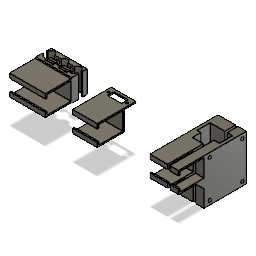
Expanded Dock v9 (Autodesk Fusion 360 design; units mm, degrees)
Autodesk Fusion 360 part; units mm, degrees
(part 1 of 2)
sketch "Sketch1" plane through (0, 0, 0) normal (1, 0, 0) x (0, 0, -1)
  line L0 (0, 0) -> (27, 0)
  line L1 (27, 0) -> (27, 60)
  line L2 (27, 60) -> (0, 60)
  line L3 (0, 60) -> (0, 0)
  dimension "d1" = 60
  dimension "d2" = 27
  constraint horizontal L0
  constraint vertical L1
  constraint horizontal L2
  constraint vertical L3
  constraint coincident L0.start L3.end
  measures "d1" distance of L0.start L2.end
  measures "d2" distance of L0.start L0.end
  measures "d70" distance of L0.end
  measures "d79" distance of L0.end
extrude "Extrude1" add sketch "Sketch1" along normal blind 2 makes body 1
sketch "Sketch2" plane through (2, 0, 0) normal (1, 0, 0) x (0, 0, -1)
  line L0 (0, 60) -> (0, 0)
  line L1 (0, 0) -> (27, 0)
  line L2 (27, 0) -> (27, 60)
  line L3 (27, 60) -> (0, 60)
  line L4 (0, 60) -> (11, 60)
  line L5 (11, 60) -> (11, 39)
  line L6 (11, 39) -> (0, 39)
  line L7 (0, 39) -> (0, 60)
  dimension "d5" = 21
  dimension "d6" = 11
  constraint horizontal L4
  constraint vertical L5
  constraint horizontal L6
  constraint vertical L7
  constraint coincident L0.start L3.end
  measures "d5" distance of L0.start L6.end
  measures "d6" distance of L0.start L4.end
extrude "Extrude2" add sketch "Sketch2" along normal blind 5 contours L0 L3 L4 L5 L6 L7 bodies 1
sketch "Sketch3" plane through (2, 0, 0) normal (1, 0, 0) x (0, 0, -1)
  line L0 (11, 60) -> (11, 39)
  line L1 (11, 39) -> (0, 39)
  line L2 (27, 0) -> (27, 60)
  line L3 (27, 60) -> (11, 60)
  line L4 (27, 0) -> (23, 0)
  line L5 (23, 0) -> (23, 20)
  line L6 (23, 20) -> (27, 20)
  line L7 (27, 20) -> (27, 0)
  line L8 (0, 0) -> (2, 0)
  line L9 (2, 0) -> (2, 20)
  line L10 (2, 20) -> (0, 20)
  line L11 (0, 20) -> (0, 0)
  dimension "d11" = 20
  dimension "d12" = 4
  dimension "d13" = 20
  dimension "d14" = 2
  constraint horizontal L4
  constraint vertical L5
  constraint horizontal L6
  constraint vertical L7
  constraint coincident L2.start L4.start
  constraint horizontal L8
  constraint vertical L9
  constraint horizontal L10
  constraint vertical L11
  constraint coincident L8.start L11.end
  measures "d11" distance of L2.start L6.end
  measures "d12" distance of L2.start L4.end
  measures "d13" distance of L8.start L10.end
  measures "d14" distance of L8.start L8.end
extrude "Extrude3" add sketch "Sketch3" along normal blind 27 bodies 1
sketch "Sketch4" plane through (0, 0, 0) normal (0, 0, 1) x (1, 0, 0)
  line L0 (0, 60) -> (0, 0)
  line L1 (0, 0) -> (29, 0)
  line L2 (29, 0) -> (29, 20)
  line L3 (29, 20) -> (2, 20)
  line L4 (2, 20) -> (2, 39)
  line L5 (2, 39) -> (7, 39)
  line L6 (7, 39) -> (7, 60)
  line L7 (7, 60) -> (0, 60)
  line L8 (0, 0) -> (29, 0)
  line L9 (29, 0) -> (29, 60)
  line L10 (29, 60) -> (0, 60)
  line L11 (0, 60) -> (0, 0)
  dimension "d17" = 29
  constraint horizontal L8
  constraint vertical L9
  constraint horizontal L10
  constraint vertical L11
  constraint coincident L0.end L1.start
  measures "d17" distance of L0.end L1.end
extrude "Extrude4" add sketch "Sketch4" along normal blind 5 bodies 1
sketch "Sketch5" plane through (0, 0, -27) normal (0, 0, -1) x (-1, 0, 0)
  line L0 (0, 0) -> (0, 60)
  line L1 (0, 60) -> (-2, 60)
  line L2 (-2, 60) -> (-2, 20)
  line L3 (-2, 20) -> (-29, 20)
  line L4 (-29, 20) -> (-29, 0)
  line L5 (-29, 0) -> (0, 0)
  line L6 (0, 0) -> (-29, 0)
  line L7 (-29, 0) -> (-29, 60)
  line L8 (-29, 60) -> (0, 60)
  line L9 (0, 60) -> (0, 0)
  dimension "d20" = 29
  constraint horizontal L6
  constraint vertical L7
  constraint horizontal L8
  constraint vertical L9
  constraint coincident L0.start L5.end
  measures "d20" distance of L0.start L4.end
extrude "Extrude5" add sketch "Sketch5" along normal blind 2 bodies 1
extrude "Extrude6" add 1 faces at (9.6667, 20, -29) along direction (0, 0, -1) blind 3 on bodies 1 bodies 1
sketch "Sketch6" plane through (29, 0, 0) normal (1, 0, 0) x (0, 0, -1)
  line L0 (-5, 0) -> (2, 0)
  line L1 (2, 0) -> (2, 20)
  line L2 (2, 20) -> (0, 20)
  line L3 (0, 20) -> (0, 60)
  line L4 (0, 60) -> (-5, 60)
  line L5 (-5, 60) -> (-5, 0)
  line L6 (32, 0) -> (-5, 0)
  line L7 (-5, 0) -> (-5, 60)
  line L8 (-5, 60) -> (32, 60)
  line L9 (32, 60) -> (32, 0)
  line L10 (32, 0) -> (32, 60)
  line L11 (23, 0) -> (27, 0)
  line L12 (27, 0) -> (27, 20)
  line L13 (27, 20) -> (23, 20)
  line L14 (23, 20) -> (23, 0)
  line L15 (27, 60) -> (32, 60)
  line L16 (32, 60) -> (32, 0)
  line L17 (32, 0) -> (27, 0)
  line L18 (27, 0) -> (27, 60)
  point P0 (23, 0)
  point P1 (27, 20)
  point P2 (27, 60)
  constraint horizontal L6
  constraint vertical L7
  constraint horizontal L8
  constraint vertical L9
  constraint coincident L4.end L5.start
  constraint coincident L6.start L10
  constraint horizontal L11
  constraint vertical L12
  constraint horizontal L13
  constraint vertical L14
  constraint coincident P1 L12.end
  constraint coincident P0 L11.start
  constraint horizontal L15
  constraint vertical L16
  constraint horizontal L17
  constraint vertical L18
  constraint coincident L6.start L9.end
  constraint coincident P2 L15.start
extrude "Extrude7" add sketch "Sketch6" along normal blind 5 separate body contours L0 L1 L2 L3 L4 L5 L6 L7 L8 | L6 L11 L12 L13 L14 L18 | L6 L8 L9 L10 L12 L15 L16 L17 L18 makes body 2 at (29, 6.6667, 1) makes body 3 at (29, 6.6667, -27.3333)
sketch "Sketch7" plane through (34, 0, 0) normal (1, 0, 0) x (0, 0, -1)
  line L0 (2, 0) -> (2, 20)
  line L1 (2, 20) -> (0, 20)
  line L2 (0, 20) -> (0, 60)
  line L3 (0, 60) -> (-5, 60)
  line L4 (-5, 60) -> (-5, 0)
  line L5 (-5, 0) -> (2, 0)
  line L6 (32, 0) -> (-5, 0)
  line L7 (-5, 0) -> (-5, 60)
  line L8 (-5, 60) -> (32, 60)
  line L9 (32, 60) -> (32, 0)
  point P0 (32, 0)
  constraint horizontal L6
  constraint vertical L7
  constraint horizontal L8
  constraint vertical L9
  constraint coincident L3.end L4.start
  constraint coincident P0 L6.start
extrude "Extrude8" add sketch "Sketch7" along normal blind 1 bodies 2 3
extrude "Extrude9" cut 2 faces at (29, 6.6667, -27.3333) (29, 6.6667, 1) along direction (-1, 0, 0) blind 1 on bodies 1 bodies 1
extrude "Extrude10" cut 2 faces at (28, 6.6667, -27.3333) (28, 6.6667, 1) along direction (-1, 0, 0) blind 5 on bodies 1 bodies 1
extrude "Extrude11" add 2 faces at (29, 6.6667, -27.3333) (29, 6.6667, 1) along direction (-1, 0, 0) blind 1 on bodies 2 bodies 2
extrude "Extrude12" add 1 faces at (34, 46.6667, -16.6667) along direction (-1, 0, 0) blind 5 on bodies 2 bodies 2
sketch "Sketch8" plane through (7, 0, 0) normal (1, 0, 0) x (0, 0, -1)
  line L0 (0, 39) -> (11, 39)
  line L1 (11, 39) -> (11, 60)
  line L2 (11, 60) -> (0, 60)
  line L3 (0, 60) -> (0, 39)
extrude "Extrude13" add sketch "Sketch8" along normal blind 17 and the other way blind -22 bodies 2
extrude "Extrude14" add 2 faces at (28, 6.6667, 1) (28, 6.6667, -27.3333) along direction (-1, 0, 0) blind 4 on bodies 2 bodies 2
extrude "Extrude15" cut 2 faces at (23, 6.6667, 1) (23, 6.6667, -27.3333) along direction (-1, 0, 0) blind 2 on bodies 1 bodies 1
extrude "Extrude16" cut 1 faces at (29, 39.6667, -21.6667) along direction (1, 0, 0) blind 2 on bodies 2 bodies 2
sketch "Sketch9" plane through (31, 0, 0) normal (-1, 0, 0) x (0, 0, 1)
  line L0 (0, 39) -> (-11, 39)
  line L1 (-11, 39) -> (-11, 60)
  line L2 (-11, 60) -> (-27, 60)
  line L3 (-27, 60) -> (-27, 20)
  line L4 (-27, 20) -> (-23, 20)
  line L5 (-23, 20) -> (-23, 0)
  line L6 (-23, 0) -> (-2, 0)
  line L7 (-2, 0) -> (-2, 20)
  line L8 (-2, 20) -> (0, 20)
  line L9 (0, 20) -> (0, 39)
  line L10 (-23, 20) -> (-2, 20)
  line L11 (-2, 20) -> (-2, 0)
  line L12 (-2, 0) -> (-23, 0)
  line L13 (-23, 0) -> (-23, 20)
  constraint horizontal L10
  constraint vertical L11
  constraint horizontal L12
  constraint vertical L13
  constraint coincident L6.end L7.start
  constraint coincident L4.end L5.start
extrude "Extrude17" cut sketch "Sketch9" against normal blind 2 contours L5 L6 L7 L10 L11 L12 L13 bodies 2
sketch "Sketch10" plane through (2, 0, 0) normal (1, 0, 0) x (0, 0, -1)
  line L0 (23, 0) -> (23, 20)
  line L1 (23, 20) -> (27, 20)
  line L2 (27, 20) -> (27, 60)
  line L3 (27, 60) -> (11, 60)
  line L4 (11, 60) -> (11, 39)
  line L5 (11, 39) -> (0, 39)
  line L6 (0, 39) -> (0, 20)
  line L7 (0, 20) -> (2, 20)
  line L8 (2, 20) -> (2, 0)
  line L9 (2, 0) -> (23, 0)
  line L10 (2, 20) -> (23, 20)
  line L11 (23, 20) -> (23, 0)
  line L12 (23, 0) -> (2, 0)
  line L13 (2, 0) -> (2, 20)
  constraint horizontal L10
  constraint vertical L11
  constraint horizontal L12
  constraint vertical L13
  constraint coincident L0.start L9.end
  constraint coincident L7.end L8.start
extrude "Extrude18" cut sketch "Sketch10" against normal blind 1 contours L0 L8 L9 L10 L11 L12 L13 bodies 1
extrude "Extrude19" add 1 faces at (0, 40, -19.6667) along direction (-1, 0, 0) blind 3 on bodies 1 bodies 1
extrude "Extrude20" cut 1 faces at (1, 13.3333, -16) along direction (-1, 0, 0) blind 1 on bodies 1 bodies 1
chamfer "Chamfer1" distance 4 angle 45 2 edges at (27.5, 20, -27) (11.5, 20, -27) on bodies 1 2
chamfer "Chamfer2" distance 2 angle 45 2 edges at (27.5, 20, 0) (11.5, 20, 0) on bodies 1 2
extrude "Extrude21" add 2 faces at (13, 40, 5) (31.3333, 40, 5) along direction (0, 0, 1) blind 2 on bodies 1 2 bodies 1 2
extrude "Extrude22" add 2 faces at (5, 40, -32) (27.6667, 40, -32) along direction (0, 0, -1) blind 2 on bodies 1 2 bodies 1 2
extrude "Extrude23" add 1 faces at (13, 40, 7) along direction (0, 0, 1) blind 4 on bodies 1 bodies 1
extrude "Extrude24" add 1 faces at (31.3333, 40, 7) along direction (0, 0, 1) blind 4 on bodies 2 bodies 2
extrude "Extrude25" add 1 faces at (5, 40, -34) along direction (0, 0, -1) blind 4 on bodies 1 bodies 1
extrude "Extrude26" add 1 faces at (27.6667, 40, -34) along direction (0, 0, -1) blind 4 on bodies 2 bodies 2
sketch "Sketch11" plane through (35, 0, 0) normal (1, 0, 0) x (0, 0, -1)
  line L0 (38, 60) -> (-11, 60)
  line L1 (-11, 60) -> (-11, 0)
  line L2 (-11, 0) -> (38, 0)
  line L3 (38, 0) -> (38, 60)
  line L4 (-11, 60) -> (0, 60)
  line L5 (0, 60) -> (0, 49)
  line L6 (0, 49) -> (-11, 49)
  line L7 (-11, 49) -> (-11, 60)
  line L8 (0, 54.5) -> (-5, 54.5)
  circle A0 centre (-5, 54.5) radius 2.35
  dimension "d69" = 11
  dimension "d70" = 11
  dimension "d71" = 4.7
  constraint horizontal L4
  constraint vertical L5
  constraint horizontal L6
  constraint vertical L7
  constraint coincident L0.end L1.start
  constraint midpoint L5 L8.start
  constraint perpendicular L5 L8
  constraint coincident L8.end A0.centre
  measures "d69" distance of L0.end L4.end
  measures "d70" distance of L0.end L6.end
  measures "d71" diameter of A0
extrude "Extrude27" cut sketch "Sketch11" against normal blind 25 contours A0 bodies 1 2
sketch "Sketch12" plane through (35, 0, 0) normal (1, 0, 0) x (0, 0, -1)
  circle A0 centre (-5, 54.5) radius 2.35
  line L0 (38, 60) -> (-11, 60)
  line L1 (-11, 60) -> (-11, 0)
  line L2 (-11, 0) -> (38, 0)
  line L3 (38, 0) -> (38, 60)
  line L4 (38, 0) -> (27, 0)
  line L5 (27, 0) -> (27, 11)
  line L6 (27, 11) -> (38, 11)
  line L7 (38, 11) -> (38, 0)
  line L8 (38, 60) -> (27, 60)
  line L9 (27, 60) -> (27, 49)
  line L10 (27, 49) -> (38, 49)
  line L11 (38, 49) -> (38, 60)
  line L12 (-11, 0) -> (0, 0)
  line L13 (0, 0) -> (0, 11)
  line L14 (0, 11) -> (-11, 11)
  line L15 (-11, 11) -> (-11, 0)
  line L16 (0, 5.5) -> (-11, 5.5)
  line L17 (27, 5.5) -> (38, 5.5)
  line L18 (32.5, 49) -> (32.5, 60)
  circle A1 centre (32.5, 54.5) radius 2.35
  circle A2 centre (32.5, 5.5) radius 2.35
  circle A3 centre (-5.5, 5.5) radius 2.35
  dimension "d74" = 11
  dimension "d75" = 11
  dimension "d76" = 11
  dimension "d77" = 11
  dimension "d78" = 11
  dimension "d79" = 11
  dimension "d80" = 4.7
  dimension "d81" = 4.7
  dimension "d82" = 4.7
  constraint horizontal L4
  constraint vertical L5
  constraint horizontal L6
  constraint vertical L7
  constraint coincident L2.end L3.start
  constraint horizontal L8
  constraint vertical L9
  constraint horizontal L10
  constraint vertical L11
  constraint coincident L0.start L3.end
  constraint horizontal L12
  constraint vertical L13
  constraint horizontal L14
  constraint vertical L15
  constraint coincident L1.end L2.start
  constraint midpoint L13 L16.start
  constraint midpoint L15 L16.end
  constraint midpoint L5 L17.start
  constraint midpoint L7 L17.end
  constraint midpoint L10 L18.start
  constraint midpoint L8 L18.end
  constraint midpoint L18 A1.centre
  constraint midpoint L17 A2.centre
  constraint midpoint L16 A3.centre
  measures "d74" distance of L2.end L6.end
  measures "d75" distance of L2.end L4.end
  measures "d76" distance of L0.start L10.end
  measures "d77" distance of L0.start L8.end
  measures "d78" distance of L1.end L12.end
  measures "d79" distance of L1.end L14.end
  measures "d80" diameter of A1
  measures "d81" diameter of A2
  measures "d82" diameter of A3
extrude "Extrude28" cut sketch "Sketch12" against normal blind 25 contours L18 A1 | L18 A1 | L17 A2 | L17 A2 | L16 A3 | L16 A3 bodies 1 2
extrude "Extrude29" cut 4 faces at (10, 52.9552, 5.1158) (10, 6.1772, 5.5585) (10, 6.0708, -33.2406) (10, 54.3859, -33.2398) along direction (-1, 0, 0) blind 8 on bodies 1 bodies 1
sketch "Sketch13" plane through (35, 0, 0) normal (1, 0, 0) x (0, 0, -1)
  circle A0 centre (-5.5, 5.5) radius 2.35
  circle A1 centre (32.5, 5.5) radius 2.35
  circle A2 centre (32.5, 54.5) radius 2.35
  circle A3 centre (-5, 54.5) radius 2.35
  line L0 (38, 60) -> (-11, 60)
  line L1 (-11, 60) -> (-11, 0)
  line L2 (-11, 0) -> (38, 0)
  line L3 (38, 0) -> (38, 60)
  circle A4 centre (-5, 54.5) radius 4.7
  circle A5 centre (32.5, 54.5) radius 4.7
  circle A6 centre (-5.5, 5.5) radius 4.7
  circle A7 centre (32.5, 5.5) radius 4.7
  dimension "d87" = 9.4
  dimension "d88" = 9.4
  dimension "d89" = 9.4
  dimension "d90" = 9.4
  constraint concentric A3 A4
  constraint concentric A2 A5
  constraint concentric A0 A6
  constraint concentric A1 A7
  measures "d87" diameter of A4
  measures "d88" diameter of A5
  measures "d89" diameter of A6
  measures "d90" diameter of A7
extrude "Extrude30" cut sketch "Sketch13" against normal blind 3.5 contours A4 | A5 | A6 | A7 bodies 2
sketch "Sketch14" plane through (0, 0, -38) normal (0, 0, -1) x (-1, 0, 0)
  line L0 (-21, 60) -> (-21, 0)
  line L1 (-21, 0) -> (3, 0)
  line L2 (3, 0) -> (3, 60)
  line L3 (3, 60) -> (-21, 60)
  line L4 (-21, 0) -> (-10, 0)
  line L5 (-10, 0) -> (-10, 11)
  line L6 (-10, 11) -> (-21, 11)
  line L7 (-21, 11) -> (-21, 0)
  line L8 (-15.5, 11) -> (-15.5, 0)
  line L9 (-10, 5.5) -> (-21, 5.5)
  line L10 (-15.5, 5.5) -> (-13.85, 5.5)
  line L11 (-13.85, 5.5) -> (-13.85, 10.3)
  line L12 (-13.85, 10.3) -> (-15.5, 10.3)
  line L13 (-15.5, 10.3) -> (-15.5, 5.5)
  line L14 (-13.85, 10.3) -> (-17.15, 10.3)
  line L15 (-17.15, 10.3) -> (-17.15, 0.7)
  line L16 (-17.15, 0.7) -> (-13.85, 0.7)
  line L17 (-13.85, 0.7) -> (-13.85, 10.3)
  point P0 (-21, 5.5)
  dimension "d93" = 11
  dimension "d94" = 11
  dimension "d95" = 4.8
  dimension "d96" = 1.65
  dimension "d97" = 9.6
  dimension "d98" = 3.3
  constraint horizontal L4
  constraint vertical L5
  constraint horizontal L6
  constraint vertical L7
  constraint coincident L0.end L1.start
  constraint midpoint L6 L8.start
  constraint midpoint L4 L8.end
  constraint midpoint L5 L9.start
  constraint coincident P0 L9.end
  constraint horizontal L10
  constraint vertical L11
  constraint horizontal L12
  constraint vertical L13
  constraint midpoint L9 L10.start
  constraint horizontal L14
  constraint vertical L15
  constraint horizontal L16
  constraint vertical L17
  measures "d93" distance of L0.end L4.end
  measures "d94" distance of L0.end L6.end
  measures "d95" distance of L10.start L12.end
  measures "d96" distance of L10.start L10.end
  measures "d97" distance of L11.end L16.end
  measures "d98" distance of L11.end L14.end
extrude "Extrude31" cut sketch "Sketch14" against normal blind 10.8 contours L8 L9 L13 L14 L15 | L8 L9 L15 L16 | L8 L9 L10 L11 L12 L13 L14 L17 | L8 L9 L10 L16 L17 bodies 1
chamfer "Chamfer3" distance 0.5 angle 45 2 edges at (15.5, 0.7, -38) (15.5, 10.3, -38) on bodies 1
sketch "Sketch15" plane through (0, 0, -38) normal (0, 0, -1) x (-1, 0, 0)
  line L0 (-13.85, 10.8) -> (-13.85, 0.2)
  line L1 (-13.85, 0.2) -> (-17.15, 0.2)
  line L2 (-17.15, 0.2) -> (-17.15, 10.8)
  line L3 (-17.15, 10.8) -> (-13.85, 10.8)
  line L4 (-21, 60) -> (-21, 0)
  line L5 (-21, 0) -> (3, 0)
  line L6 (3, 0) -> (3, 60)
  line L7 (3, 60) -> (-21, 60)
  line L8 (-21, 60) -> (-10, 60)
  line L9 (-10, 60) -> (-10, 49)
  line L10 (-10, 49) -> (-21, 49)
  line L11 (-21, 49) -> (-21, 60)
  line L12 (-15.5, 60) -> (-15.5, 49)
  line L13 (-15.5, 54.5) -> (-13.85, 54.5)
  line L14 (-13.85, 54.5) -> (-13.85, 49.7)
  line L15 (-13.85, 49.7) -> (-15.5, 49.7)
  line L16 (-15.5, 49.7) -> (-15.5, 54.5)
  line L17 (-13.85, 49.7) -> (-17.15, 49.7)
  line L18 (-17.15, 49.7) -> (-17.15, 59.5)
  line L19 (-17.15, 59.5) -> (-13.85, 59.5)
  line L20 (-13.85, 59.5) -> (-13.85, 49.7)
  dimension "d102" = 11
  dimension "d103" = 11
  dimension "d104" = 4.8
  dimension "d105" = 1.65
  dimension "d106" = 9.8
  dimension "d107" = 3.3
  constraint horizontal L8
  constraint vertical L9
  constraint horizontal L10
  constraint vertical L11
  constraint coincident L4.start L7.end
  constraint midpoint L8 L12.start
  constraint midpoint L10 L12.end
  constraint horizontal L13
  constraint vertical L14
  constraint horizontal L15
  constraint vertical L16
  constraint midpoint L12 L13.start
  constraint horizontal L17
  constraint vertical L18
  constraint horizontal L19
  constraint vertical L20
  measures "d102" distance of L4.start L8.end
  measures "d103" distance of L4.start L10.end
  measures "d104" distance of L13.start L15.end
  measures "d105" distance of L13.start L13.end
  measures "d106" distance of L14.end L19.end
  measures "d107" distance of L14.end L17.end
extrude "Extrude32" cut sketch "Sketch15" against normal blind 10.8 contours L12 L13 L19 L20 | L12 L16 L17 L18 L19 | L12 L13 L14 L15 L16 L17 L20 bodies 1
chamfer "Chamfer4" distance 0.5 angle 45 2 edges at (15.5, 59.5, -38) (15.5, 49.7, -38) on bodies 1
sketch "Sketch16" plane through (0, 0, 11) normal (0, 0, 1) x (1, 0, 0)
  line L0 (21, 0) -> (21, 60)
  line L1 (21, 60) -> (-3, 60)
  line L2 (-3, 60) -> (-3, 0)
  line L3 (-3, 0) -> (21, 0)
  line L4 (21, 60) -> (10, 60)
  line L5 (10, 60) -> (10, 49)
  line L6 (10, 49) -> (21, 49)
  line L7 (21, 49) -> (21, 60)
  line L8 (10, 54.5) -> (21, 54.5)
  line L9 (21, 0) -> (10, 0)
  line L10 (10, 0) -> (10, 11)
  line L11 (10, 11) -> (21, 11)
  line L12 (21, 11) -> (21, 0)
  line L13 (10, 5.5) -> (21, 5.5)
  line L14 (15.5, 5.5) -> (17.15, 5.5)
  line L15 (17.15, 5.5) -> (17.15, 10.3)
  line L16 (17.15, 10.3) -> (15.5, 10.3)
  line L17 (15.5, 10.3) -> (15.5, 5.5)
  line L18 (17.15, 10.3) -> (13.85, 10.3)
  line L19 (13.85, 10.3) -> (13.85, 0.7)
  line L20 (13.85, 0.7) -> (17.15, 0.7)
  line L21 (17.15, 0.7) -> (17.15, 10.3)
  line L22 (15.5, 54.5) -> (17.15, 54.5)
  line L23 (17.15, 54.5) -> (17.15, 59.3)
  line L24 (17.15, 59.3) -> (15.5, 59.3)
  line L25 (15.5, 59.3) -> (15.5, 54.5)
  line L26 (17.15, 59.3) -> (13.85, 59.3)
  line L27 (13.85, 59.3) -> (13.85, 49.7)
  line L28 (13.85, 49.7) -> (17.15, 49.7)
  line L29 (17.15, 49.7) -> (17.15, 59.3)
  point P0 (21, 54.5)
  point P1 (21, 5.5)
  point P2 (13.85, 49.7)
  dimension "d111" = 11
  dimension "d112" = 11
  dimension "d113" = 11
  dimension "d114" = 11
  dimension "d115" = 4.8
  dimension "d116" = 1.65
  dimension "d117" = 9.6
  dimension "d118" = 3.3
  dimension "d119" = 4.8
  constraint horizontal L4
  constraint vertical L5
  constraint horizontal L6
  constraint vertical L7
  constraint coincident L0.end L1.start
  constraint midpoint L5 L8.start
  constraint coincident P0 L8.end
  constraint horizontal L9
  constraint vertical L10
  constraint horizontal L11
  constraint vertical L12
  constraint coincident L0.start L3.end
  constraint midpoint L10 L13.start
  constraint coincident P1 L13.end
  constraint horizontal L14
  constraint vertical L15
  constraint horizontal L16
  constraint vertical L17
  constraint midpoint L13 L14.start
  constraint horizontal L18
  constraint vertical L19
  constraint horizontal L20
  constraint vertical L21
  constraint horizontal L22
  constraint vertical L23
  constraint horizontal L24
  constraint vertical L25
  constraint midpoint L8 L22.start
  constraint horizontal L26
  constraint vertical L27
  constraint horizontal L28
  constraint vertical L29
  constraint coincident P2 L27.end
  measures "d111" distance of L0.end L4.end
  measures "d112" distance of L0.end L6.end
  measures "d113" distance of L0.start L9.end
  measures "d114" distance of L0.start L11.end
  measures "d115" distance of L14.start L16.end
  measures "d116" distance of L14.start L14.end
  measures "d117" distance of L15.end L20.end
  measures "d118" distance of L15.end L18.end
  measures "d119" distance of L22.start L24.end
extrude "Extrude33" cut sketch "Sketch16" against normal blind 10.8 contours L13 L14 L19 L20 L21 | L13 L14 L15 L16 L17 L18 L21 | L13 L17 L18 L19 | L8 L22 L27 L28 L29 | L8 L22 L23 L24 L25 L26 L29 | L8 L25 L26 L27 bodies 1
move_face "MoveFace1" to x (1, 0, 0) y (0, 1, 0) z (0, 0, 1) at (0, 0, -3) 18 faces at (14.95, 56.2333, -27.2) (14.95, 49.5334, -37.6667) (14.95, 49.7, -34.0667) (16.05, 59.5, -30.6334) (16.05, 59.6666, -37.6667) (5.95, 53.6963, -30.2917) (13.85, 54.5667, -28.1833) (18.4333, 53.6963, -30.2917) (17.15, 54.5667, -28.1833) (17.15, 5.5, -28.1833) (19.7167, 5.266, -34.8383) (16.05, 0.3667, -37.8333) (16.05, 0.7, -34.0667) (14.95, 10.6333, -37.8333) (14.95, 10.3, -34.0667) (13.85, 5.5, -28.1833) (5.95, 5.3829, -34.8471) (2.6167, 23.6, -38) on bodies 1
move_face "MoveFace2" to x (1, 0, 0) y (0, 1, 0) z (0, 0, 1) at (0, 0, -3) 7 faces at (27.6667, 40, -38) (32.6667, 5.032, -37.1766) (31.5, 5.1498, -36.3904) (29, 5.3829, -34.8471) (26.5, 53.5872, -30.3345) (31.5, 54.1498, -36.3904) (32.6667, 54.032, -37.1766) on bodies 2
move_face "MoveFace3" to x (1, 0, 0) y (0, 1, 0) z (0, 0, 1) at (0, 0, 3) 7 faces at (31.3333, 40, 11) (32.6667, 5.968, 0.8234) (31.5, 5.8502, 1.6096) (26.5, 5.266, 3.1617) (29, 55.6239, 2.9362) (31.5, 54.7335, 1.1008) (33.8333, 54.7343, 0.3058) on bodies 2
move_face "MoveFace4" to x (1, 0, 0) y (0, 1, 0) z (0, 0, 1) at (0, 0, 3) 15 faces at (13.85, 5.5, 9.95) (9.9, 5.266, 3.1617) (16.05, 10.3, 3.8) (18.4333, 5.3829, 3.1529) (17.15, 5.5, 9.95) (14.95, 0.7, 7.4) (14.95, 49.7, 7.4) (16.05, 56.1, 0.2) (17.15, 54.5, 9.7833) (19.7167, 54.734, 2.6617) (16.05, 59.3, 3.8) (13.85, 54.5, 9.7833) (9.9, 55.6239, 2.9362) (14.95, 7.1, 0.2) (2.6167, 23.4333, 11) on bodies 1
extrude "Extrude34" cut 2 faces at (3.6667, 53, -11) (28.6667, 46, -11) along direction (0, 0, 1) blind 1 on bodies 1 2 bodies 1 2
extrude "Extrude35" cut 1 faces at (16.3333, 40.3332, 0) along direction (0, 0, 1) blind 1 on bodies 1 bodies 1
extrude "Extrude36" add 1 faces at (8.3333, 60, 9.6667) along direction (0, 1, 0) blind 2 on bodies 1 bodies 1
extrude "Extrude37" add 1 faces at (30.1667, 60, 8.6633) along direction (0, 1, 0) blind 2 on bodies 2 bodies 2
extrude "Extrude38" add 1 faces at (30.6667, 0, 8.6667) along direction (0, -1, 0) blind 2 on bodies 2 bodies 2
extrude "Extrude39" add 1 faces at (6, 0, 8.6667) along direction (0, -1, 0) blind 2 on bodies 1 bodies 1
sketch "Sketch17" plane through (-3, 0, 0) normal (-1, 0, 0) x (0, 0, 1)
  line L0 (-41, 62) -> (-41, -2)
  line L1 (-41, -2) -> (14, -2)
  line L2 (14, -2) -> (14, 62)
  line L3 (14, 62) -> (-41, 62)
  line L4 (14, 62) -> (45, 62)
  line L5 (45, 62) -> (45, 60)
  line L6 (45, 60) -> (14, 60)
  line L7 (14, 60) -> (14, 62)
  line L8 (45, 62) -> (47, 62)
  line L9 (47, 62) -> (47, 56)
  line L10 (47, 56) -> (45, 56)
  line L11 (45, 56) -> (45, 62)
  line L12 (14, 60) -> (14, 37)
  line L13 (14, 37) -> (45, 37)
  line L14 (45, 37) -> (45, 35)
  line L15 (45, 35) -> (14, 35)
  line L16 (14, 35) -> (14, 37)
  line L17 (45, 35) -> (47, 35)
  line L18 (47, 35) -> (47, 41)
  line L19 (47, 41) -> (45, 41)
  line L20 (45, 41) -> (45, 35)
  dimension "d134" = 31
  dimension "d135" = 2
  dimension "d136" = 2
  dimension "d137" = 6
  dimension "d138" = 23
  dimension "d139" = 31
  dimension "d140" = 2
  dimension "d141" = 6
  dimension "d142" = 2
  constraint horizontal L4
  constraint vertical L5
  constraint horizontal L6
  constraint vertical L7
  constraint coincident L2.end L3.start
  constraint horizontal L8
  constraint vertical L9
  constraint horizontal L10
  constraint vertical L11
  constraint perpendicular L6 L12
  constraint horizontal L13
  constraint vertical L14
  constraint horizontal L15
  constraint vertical L16
  constraint horizontal L17
  constraint vertical L18
  constraint horizontal L19
  constraint vertical L20
  measures "d134" distance of L2.end L4.end
  measures "d135" distance of L2.end L6.end
  measures "d136" distance of L4.end L8.end
  measures "d137" distance of L4.end L10.end
  measures "d138" distance of L6.end L12.end
  measures "d139" distance of L12.end L13.end
  measures "d140" distance of L12.end L15.end
  measures "d141" distance of L14.end L19.end
  measures "d142" distance of L14.end L17.end
extrude "Extrude40" add sketch "Sketch17" against normal blind 24 contours L2 L4 L5 L6 L7 L11 | L5 L8 L9 L10 L11 | L2 L13 L14 L15 L16 L20 | L14 L17 L18 L19 L20 bodies 1
chamfer "Chamfer5" distance 10 angle 45 1 edges at (9, 35, 14) on bodies 1
sketch "Sketch18" plane through (35, 0, 0) normal (1, 0, 0) x (0, 0, -1)
  circle A0 centre (-8.5, 5.5) radius 4.7
  circle A1 centre (-8, 54.5) radius 4.7
  circle A2 centre (35.5, 5.5) radius 4.7
  circle A3 centre (35.5, 54.5) radius 4.7
  line L0 (-14, 62) -> (-14, -2)
  line L1 (-14, -2) -> (41, -2)
  line L2 (41, -2) -> (41, 62)
  line L3 (41, 62) -> (-14, 62)
  line L4 (-14, 62) -> (-45, 62)
  line L5 (-45, 62) -> (-45, 60)
  line L6 (-45, 60) -> (-14, 60)
  line L7 (-14, 60) -> (-14, 62)
  line L8 (-45, 56) -> (-47, 56)
  line L9 (-47, 56) -> (-47, 62)
  line L10 (-47, 62) -> (-45, 62)
  line L11 (-45, 62) -> (-45, 56)
  line L12 (-47, 41) -> (-45, 41)
  line L13 (-45, 41) -> (-45, 35)
  line L14 (-45, 35) -> (-47, 35)
  line L15 (-47, 35) -> (-47, 41)
  line L16 (-47, 35) -> (-24, 35)
  line L17 (-45, 35) -> (-14, 35)
  line L18 (-14, 35) -> (-14, 37)
  line L19 (-14, 37) -> (-45, 37)
  line L20 (-45, 37) -> (-45, 35)
  point P0 (-45, 60)
  point P1 (-45, 56)
  point P2 (-47, 62)
  point P3 (-47, 41)
  point P4 (-14, 37)
  constraint horizontal L4
  constraint vertical L5
  constraint horizontal L6
  constraint vertical L7
  constraint coincident P0 L5.end
  constraint coincident L0.start L3.end
  constraint horizontal L8
  constraint vertical L9
  constraint horizontal L10
  constraint vertical L11
  constraint coincident P2 L9.end
  constraint coincident P1 L8.start
  constraint horizontal L12
  constraint vertical L13
  constraint horizontal L14
  constraint vertical L15
  constraint coincident L13.end L16
  constraint coincident P3 L12.start
  constraint horizontal L17
  constraint vertical L18
  constraint horizontal L19
  constraint vertical L20
  constraint coincident P4 L18.end
extrude "Extrude41" add sketch "Sketch18" against normal blind 11 contours L0 L4 L5 L6 L7 L11 | L5 L8 L9 L10 L11 | L0 L13 L16 L17 L18 L19 L20 | L12 L13 L14 L15 L16 L20 bodies 2
chamfer "Chamfer6" distance 10 angle 45 1 edges at (29.5, 35, 14) on bodies 2
delete_face "DeleteFace1" 1 faces at (29, 54.734, 5.6617) on bodies 2
delete_face "DeleteFace2" 1 faces at (31.5, 55.6415, 6.5189) on bodies 2
delete_face "DeleteFace3" 1 faces at (27.6667, 54.032, 3.3234) on bodies 2
delete_face "DeleteFace4" 1 faces at (29, 54.734, -37.8383) on bodies 2
delete_face "DeleteFace5" 1 faces at (31.5, 55.9584, -34.9276) on bodies 2
delete_face "DeleteFace6" 1 faces at (27.6667, 54.032, -40.1766) on bodies 2
delete_face "DeleteFace7" 6 faces at (29, 5.734, -37.8383) (31.5, 5.7335, -39.3992) (33.8333, 5.7343, -40.1942) (29, 5.734, 6.1617) (31.5, 5.7335, 4.6008) (32.6667, 5.968, 3.8234) on bodies 2
delete_face "DeleteFace8" 7 faces at (19.7167, 5.734, 6.1617) (17.15, 5.5, 12.95) (16.05, 7.1, 3.2) (16.05, 10.3, 6.8) (13.85, 5.5, 12.95) (9.9, 5.6171, 6.1529) (14.95, 0.7, 10.4) on bodies 1
delete_face "DeleteFace9" 7 faces at (13.85, 54.5, 12.7833) (5.95, 54.6171, 5.6529) (18.4333, 55.6239, 10.0638) (16.05, 59.3, 10.4) (17.15, 54.5, 12.7833) (16.05, 56.1, 3.2) (16.05, 49.7, 10.4) on bodies 1
delete_face "DeleteFace10" 9 faces at (5.95, 56.0106, -37.3002) (19.7167, 54.6171, -33.1529) (14.95, 49.5334, -40.6667) (14.95, 49.7, -37.0667) (13.85, 54.5667, -31.1833) (14.95, 59.5, -37.0667) (14.95, 59.8333, -40.8334) (14.95, 56.2333, -30.2) (17.15, 54.5667, -31.1833) on bodies 1
delete_face "DeleteFace11" 9 faces at (16.05, 7.1, -27.2) (17.15, 5.5, -29.1833) (19.7167, 5.734, -37.8383) (16.05, 10.3, -31.6333) (16.05, 10.6333, -40.8333) (9.9, 5.6171, -37.8471) (13.85, 5.5, -29.1833) (16.05, 0.7, -31.6333) (16.05, 0.5333, -40.6667) on bodies 1
move_face "MoveFace5" by (0, -5, 0) 8 faces at (8.3333, 62, 31.6667) (30, 62, 28) (31.3333, 60, 34.6667) (13, 60, 34.6667) (5, 60, 47) (5, 56, 46.3333) (31.3333, 58, 47) (31.3333, 56, 45.6667) on bodies 1 2
move_face "MoveFace6" by (0, -5, 0) 8 faces at (27.6667, 35, 31.6667) (13, 35, 39.3333) (5, 28.3333, 17.3333) (27.6667, 28.3333, 17.3333) (27.6667, 37, 24.3333) (31.3333, 41, 46.3333) (13, 37, 34.6667) (13, 41, 46.3333) on bodies 1 2
sketch "Sketch19" plane through (35, 0, 0) normal (1, 0, 0) x (0, 0, -1)
  line L0 (-14, 20) -> (-14, -2)
  line L1 (-14, -2) -> (41, -2)
  line L2 (41, -2) -> (41, 57)
  line L3 (41, 57) -> (-47, 57)
  line L4 (-47, 57) -> (-47, 51)
  line L5 (-47, 51) -> (-45, 51)
  line L6 (-45, 51) -> (-45, 55)
  line L7 (-45, 55) -> (-14, 55)
  line L8 (-14, 55) -> (-14, 32)
  line L9 (-14, 32) -> (-45, 32)
  line L10 (-45, 32) -> (-45, 36)
  line L11 (-45, 36) -> (-47, 36)
  line L12 (-47, 36) -> (-47, 30)
  line L13 (-47, 30) -> (-24, 30)
  line L14 (-24, 30) -> (-14, 20)
  line L15 (41, 57) -> (30, 57)
  line L16 (30, 57) -> (30, 46)
  line L17 (30, 46) -> (41, 46)
  line L18 (41, 46) -> (41, 57)
  line L19 (35.5, 57) -> (35.5, 46)
  circle A0 centre (35.5, 51.5) radius 2.05
  line L20 (41, -2) -> (30, -2)
  line L21 (30, -2) -> (30, 9)
  line L22 (30, 9) -> (41, 9)
  line L23 (41, 9) -> (41, -2)
  line L24 (30, 3.5) -> (41, 3.5)
  circle A1 centre (35.5, 3.5) radius 2.05
  line L25 (-1, 57) -> (-12, 57)
  line L26 (-12, 57) -> (-12, 46)
  line L27 (-12, 46) -> (-1, 46)
  line L28 (-1, 46) -> (-1, 57)
  line L29 (-12, 51.5) -> (-1, 51.5)
  line L30 (-12, 46) -> (-1, 46)
  line L31 (-1, 46) -> (-1, -2)
  line L32 (-1, -2) -> (-12, -2)
  line L33 (-12, -2) -> (-12, 46)
  line L34 (-12, -2) -> (-1, -2)
  line L35 (-1, -2) -> (-1, 9)
  line L36 (-1, 9) -> (-12, 9)
  line L37 (-12, 9) -> (-12, -2)
  line L38 (-12, 3.5) -> (-1, 3.5)
  circle A2 centre (-6.5, 3.5) radius 2.05
  circle A3 centre (-6.5, 51.5) radius 2.05
  point P0 (-1, 57)
  dimension "d153" = 11
  dimension "d154" = 11
  dimension "d155" = 4.1
  dimension "d156" = 11
  dimension "d157" = 11
  dimension "d158" = 4.1
  dimension "d159" = 11
  dimension "d160" = 11
  dimension "d161" = 11
  dimension "d162" = 11
  dimension "d163" = 4.1
  dimension "d164" = 4.1
  constraint horizontal L15
  constraint vertical L16
  constraint horizontal L17
  constraint vertical L18
  constraint coincident L2.end L3.start
  constraint midpoint L15 L19.start
  constraint midpoint L17 L19.end
  constraint midpoint L19 A0.centre
  constraint horizontal L20
  constraint vertical L21
  constraint horizontal L22
  constraint vertical L23
  constraint coincident L1.end L2.start
  constraint midpoint L21 L24.start
  constraint midpoint L23 L24.end
  constraint midpoint L24 A1.centre
  constraint horizontal L25
  constraint vertical L26
  constraint horizontal L27
  constraint vertical L28
  constraint coincident P0 L25.start
  constraint midpoint L26 L29.start
  constraint midpoint L28 L29.end
  constraint horizontal L30
  constraint vertical L31
  constraint horizontal L32
  constraint vertical L33
  constraint horizontal L34
  constraint vertical L35
  constraint horizontal L36
  constraint vertical L37
  constraint midpoint L37 L38.start
  constraint midpoint L35 L38.end
  constraint midpoint L38 A2.centre
  constraint midpoint L29 A3.centre
  measures "d153" distance of L2.end L15.end
  measures "d154" distance of L2.end L17.end
  measures "d155" diameter of A0
  measures "d156" distance of L1.end L22.end
  measures "d157" distance of L1.end L20.end
  measures "d158" diameter of A1
  measures "d159" distance of P0 L25.end
  measures "d160" distance of P0 L27.end
  measures "d161" distance of L26.end L27.end
  measures "d162" distance of L32.end L36.end
  measures "d163" diameter of A2
  measures "d164" diameter of A3
extrude "Extrude44" cut sketch "Sketch19" against normal blind 104 contours L38 A2 | L38 A2 | L24 A1 | L24 A1 | L29 A3 | L29 A3 | L19 A0 | L19 A0 bodies 1 2
extrude "Extrude42" cut 1 faces at (-3, 29, -18.1479) along direction (1, 0, 0) blind 2 on bodies 1 bodies 1
extrude "Extrude43" add 1 faces at (-1, 29, -18.1479) along direction (-1, 0, 0) blind 1 on bodies 1 bodies 1
sketch "Sketch20" plane through (-2, 0, 0) normal (-1, 0, 0) x (0, 0, 1)
  circle A0 centre (-35.5, 51.5) radius 2.05
  circle A1 centre (-35.5, 3.5) radius 2.05
  circle A2 centre (6.5, 51.5) radius 2.05
  circle A3 centre (6.5, 3.5) radius 2.05
  line L0 (14, 32) -> (14, 55)
  line L1 (14, 55) -> (45, 55)
  line L2 (45, 55) -> (45, 51)
  line L3 (45, 51) -> (47, 51)
  line L4 (47, 51) -> (47, 57)
  line L5 (47, 57) -> (-41, 57)
  line L6 (-41, 57) -> (-41, -2)
  line L7 (-41, -2) -> (14, -2)
  line L8 (14, -2) -> (14, 20)
  line L9 (14, 20) -> (24, 30)
  line L10 (24, 30) -> (47, 30)
  line L11 (47, 30) -> (47, 36)
  line L12 (47, 36) -> (45, 36)
  line L13 (45, 36) -> (45, 32)
  line L14 (45, 32) -> (14, 32)
  line L15 (47, 30) -> (12, 30)
  line L16 (12, 30) -> (12, 57)
  line L17 (12, 57) -> (47, 57)
  line L18 (47, 57) -> (47, 30)
  constraint horizontal L15
  constraint vertical L16
  constraint horizontal L17
  constraint vertical L18
  constraint coincident L5 L16.end
  constraint coincident L10.end L11.start
extrude "Extrude45" add sketch "Sketch20" along normal blind 100 and the other way blind -65 separate body contours L0 L1 L2 L3 L4 L5 L10 L11 L12 L13 L14 L15 L16 L17 L18 makes body 4
sketch "Sketch21" plane through (0, 57, 0) normal (0, 1, 0) x (-1, 0, 0)
  line L0 (67, 47) -> (67, 12)
  line L1 (67, 12) -> (102, 12)
  line L2 (102, 12) -> (102, 47)
  line L3 (102, 47) -> (67, 47)
  line L4 (102, 12) -> (67, 12)
  line L5 (67, 12) -> (67, -3)
  line L6 (67, -3) -> (102, -3)
  line L7 (102, -3) -> (102, 12)
  line L8 (102, 4.5) -> (98, 4.5)
  circle A0 centre (98, 4.5) radius 1.5
  line L9 (67, 4.5) -> (71, 4.5)
  circle A1 centre (71, 4.5) radius 1.5
  line L10 (67, 4.5) -> (67.5398, 4.5)
  line L11 (67, 4.5) -> (67.5398, 4.5)
  line L12 (67, 4.5) -> (74, 4.5)
  line L13 (102, 4.5) -> (95, 4.5)
  line L14 (95, 4.5) -> (95, 0.4)
  line L15 (74, 4.5) -> (74, 8.6)
  line L16 (74, 8.6) -> (95, 8.6)
  line L17 (95, 8.6) -> (95, 0.4)
  line L18 (95, 0.4) -> (74, 0.4)
  line L19 (74, 0.4) -> (74, 8.6)
  dimension "d171" = 15
  dimension "d172" = 4
  dimension "d173" = 3
  dimension "d174" = 4
  dimension "d175" = 3
  dimension "d176" = 7
  dimension "d177" = 7
  dimension "d178" = 4.1
  dimension "d179" = 4.1
  constraint horizontal L4
  constraint vertical L5
  constraint horizontal L6
  constraint vertical L7
  constraint coincident L1.end L2.start
  constraint midpoint L7 L8.start
  constraint perpendicular L7 L8
  constraint coincident L8.end A0.centre
  constraint midpoint L5 L9.start
  constraint perpendicular L5 L9
  constraint coincident L9.end A1.centre
  constraint coincident L9 L10.end
  constraint parallel L9 L12
  constraint perpendicular L7 L13
  constraint perpendicular L13 L14
  constraint perpendicular L12 L15
  constraint horizontal L16
  constraint vertical L17
  constraint horizontal L18
  constraint vertical L19
  measures "d171" distance of L1.end L6.end
  measures "d172" distance of L8.start L8.end
  measures "d173" diameter of A0
  measures "d174" distance of L9.start L9.end
  measures "d175" diameter of A1
  measures "d176" distance of L9.start L12.end
  measures "d177" distance of L8.start L13.end
  measures "d178" distance of L13.end L14.end
  measures "d179" distance of L12.end L15.end
extrude "Extrude46" add sketch "Sketch21" against normal blind 4 contours L1 L4 L5 L7 L8 A0 L9 A1 L10 L11 L12 L13 L15 L16 L17 L19 | L5 L6 L7 L8 A0 L9 A1 L10 L11 L12 L13 L14 L17 L18 L19 bodies 4
extrude "Extrude47" cut 1 faces at (-81, 53, -1.8667) along direction (0, 1, 0) blind 2 on bodies 4 bodies 4
move_face "MoveFace7" to x (1, 0, 0) y (0, 1, 0) z (0, 0, 1) at (-3, 0, 0) 3 faces at (-74, 55.6667, 3.1333) (-72.4925, 56.3333, 4.6494) (-67, 56.3333, 34.6667) on bodies 4
sketch "Sketch22" plane through (-102, 0, 0) normal (-1, 0, 0) x (0, 0, 1)
  line L0 (-3, 55) -> (12, 55)
  line L1 (12, 55) -> (12, 30)
  line L2 (12, 30) -> (47, 30)
  line L3 (47, 30) -> (47, 36)
  line L4 (47, 36) -> (45, 36)
  line L5 (45, 36) -> (45, 32)
  line L6 (45, 32) -> (14, 32)
  line L7 (14, 32) -> (14, 55)
  line L8 (14, 55) -> (45, 55)
  line L9 (45, 55) -> (45, 51)
  line L10 (45, 51) -> (47, 51)
  line L11 (47, 51) -> (47, 57)
  line L12 (47, 57) -> (-3, 57)
  line L13 (-3, 57) -> (-3, 55)
  line L14 (47, 30) -> (12, 30)
  line L15 (12, 30) -> (12, 57)
  line L16 (12, 57) -> (47, 57)
  line L17 (47, 57) -> (47, 30)
  constraint horizontal L14
  constraint vertical L15
  constraint horizontal L16
  constraint vertical L17
  constraint coincident L12 L15.end
  constraint coincident L2.end L3.start
extrude "Extrude48" add sketch "Sketch22" along normal blind 43 and the other way blind -35 separate body contours L1 L2 L3 L4 L5 L6 L7 L8 L9 L10 L11 L12 L14 L15 L16 L17 makes body 5
extrude "Extrude49" add 1 faces at (-145, 56.3333, 24.3333) along direction (-1, 0, 0) blind 38.5 on bodies 5 bodies 5
sketch "Sketch23" plane through (0, 0, 12) normal (0, 0, -1) x (-1, 0, 0)
  line L0 (137, 57) -> (137, 30)
  line L1 (137, 30) -> (183.5, 30)
  line L2 (183.5, 30) -> (183.5, 57)
  line L3 (183.5, 57) -> (137, 57)
  line L4 (137, 57) -> (183.5, 57)
  line L5 (183.5, 57) -> (183.5, 59)
  line L6 (183.5, 59) -> (137, 59)
  line L7 (137, 59) -> (137, 57)
  line L8 (137, 30) -> (183.5, 30)
  line L9 (183.5, 30) -> (183.5, 28)
  line L10 (183.5, 28) -> (137, 28)
  line L11 (137, 28) -> (137, 30)
  dimension "d190" = 2
  dimension "d191" = 2
  constraint horizontal L4
  constraint vertical L5
  constraint horizontal L6
  constraint vertical L7
  constraint coincident L0.start L3.end
  constraint horizontal L8
  constraint vertical L9
  constraint horizontal L10
  constraint vertical L11
  constraint coincident L0.end L1.start
  measures "d190" distance of L0.start L6.end
  measures "d191" distance of L0.end L10.end
extrude "Extrude50" add sketch "Sketch23" along normal blind 12 separate body contours L3 L4 L5 L6 L7 | L1 L8 L9 L10 L11 makes body 6 at (-168, 59, 8) makes body 7 at (-152.5, 30, 8)
extrude "Extrude51" add 1 faces at (-152.5, 39, 12) along direction (0, 0, -1) blind 2 on bodies 5 bodies 5 6 7
extrude "Extrude52" add 1 faces at (-152.5, 58.3333, 0) along direction (0, 0, -1) blind 2 on bodies 5 bodies 5
extrude "Extrude53" add 1 faces at (-152.5, 28.6667, 0) along direction (0, 0, -1) blind 2 on bodies 5 bodies 5
chamfer "Chamfer7" distance 2 angle 45 1 edges at (-160.25, 57, 12) on bodies 5
chamfer "Chamfer8" distance 2 angle 45 1 edges at (-160.25, 30, 12) on bodies 5
sketch "Sketch24" plane through (0, 59, 0) normal (0, 1, 0) x (-1, 0, 0)
  line L0 (183.5, 12) -> (137, 12)
  line L1 (137, 12) -> (137, -2)
  line L2 (137, -2) -> (183.5, -2)
  line L3 (183.5, -2) -> (183.5, 12)
  line L4 (183.5, 12) -> (183.5, 11.9)
  line L5 (183.5, -2) -> (183.5, 10)
  line L6 (183.5, 4) -> (181.7, 4)
  line L7 (137, -2) -> (137, 10)
  line L8 (137, 4) -> (138.8, 4)
  line L9 (160.25, -2) -> (160.25, -0.2)
  line L10 (160.25, -0.2) -> (160.25, 8.2)
  line L11 (181.7, 4) -> (173.3, 4)
  line L12 (138.8, 4) -> (147.2, 4)
  circle A0 centre (177.5, 4) radius 4.2
  circle A1 centre (160.25, 4) radius 4.2
  circle A2 centre (143, 4) radius 4.2
  dimension "d202" = 1.8
  dimension "d203" = 12
  dimension "d204" = 1.8
  dimension "d205" = 1.8
  dimension "d206" = 8.4
  dimension "d207" = 8.4
  dimension "d208" = 8.4
  constraint coincident L0.start L3.end
  constraint coincident L3 L4.end
  constraint perpendicular L0 L4
  constraint coincident L2.end L3.start
  constraint coincident L3 L5.end
  constraint perpendicular L0 L5
  constraint midpoint L5 L6.start
  constraint perpendicular L5 L6
  constraint coincident L1.end L2.start
  constraint perpendicular L2 L7
  constraint midpoint L7 L8.start
  constraint perpendicular L7 L8
  constraint midpoint L2 L9.start
  constraint perpendicular L2 L9
  constraint parallel L9 L10
  constraint horizontal L11
  constraint parallel L8 L12
  constraint midpoint L11 A0.centre
  constraint coincident L11.end A0
  constraint midpoint L10 A1.centre
  constraint coincident L10.end A1
  constraint midpoint L12 A2.centre
  constraint coincident L12.end A2
  measures "d202" distance of L6.start L6.end
  measures "d203" distance of L1.end L7.end
  measures "d204" distance of L8.start L8.end
  measures "d205" distance of L9.start L9.end
  measures "d206" distance of L9.end L10.end
  measures "d207" distance of L6.end L11.end
  measures "d208" distance of L8.end L12.end
extrude "Extrude54" cut sketch "Sketch24" against normal blind 31 contours L10 A1 | L10 A1 | L11 A0 | L11 A0 | L12 A2 | L12 A2 bodies 5
extrude "Extrude55" cut 2 faces at (-168, 28.0001, 12) (-160.3546, 28, 10.7294) along direction (0, 1, 0) blind 1 on bodies 5 bodies 5
extrude "Extrude56" cut 1 faces at (-152.5, 28.3337, 12) along direction (0, 0, 1) blind 2 on bodies 5 bodies 5
extrude "Extrude57" cut 2 faces at (-168, 58.9997, 12) (-160.3546, 59, 10.7294) along direction (0, -1, 0) blind 1 on bodies 5 bodies 5
extrude "Extrude58" cut 1 faces at (-168, 58.6663, 12) along direction (0, 0, 1) blind 7 on bodies 5 bodies 5
extrude "Extrude59" add 2 faces at (-152.5, 57.6667, -2) (-152.5, 29.3333, -2) along direction (0, 0, -1) blind 10 on bodies 5 bodies 5
sketch "Sketch25" plane through (0, 58, 0) normal (0, 1, 0) x (-1, 0, 0)
  circle A0 centre (160.25, 4) radius 4.2
  circle A1 centre (177.5, 4) radius 4.2
  circle A2 centre (143, 4) radius 4.2
  line L0 (137, 13) -> (137, -12)
  line L1 (137, -12) -> (183.5, -12)
  line L2 (183.5, -12) -> (183.5, 13)
  line L3 (183.5, 13) -> (137, 13)
  line L4 (137, -12) -> (137, -2)
  line L5 (183.5, -12) -> (183.5, -2)
  line L6 (183.5, -7) -> (137, -7)
  line L7 (137, -7) -> (147, -7)
  line L8 (183.5, -7) -> (173.5, -7)
  circle A3 centre (173.5, -7) radius 4
  circle A4 centre (147, -7) radius 4
  circle A5 centre (147, -7) radius 2
  circle A6 centre (173.5, -7) radius 2
  dimension "d221" = 10
  dimension "d222" = 10
  dimension "d223" = 10
  dimension "d224" = 10
  dimension "d225" = 8
  dimension "d226" = 8
  dimension "d227" = 4
  dimension "d228" = 4
  constraint coincident L0.end L1.start
  constraint perpendicular L1 L4
  constraint coincident L1.end L2.start
  constraint perpendicular L1 L5
  constraint midpoint L5 L6.start
  constraint midpoint L4 L6.end
  constraint perpendicular L4 L7
  constraint perpendicular L2 L8
  constraint coincident L8.end A3.centre
  constraint coincident L7.end A4.centre
  constraint concentric A3 A6
  measures "d221" distance of L0.end L4.end
  measures "d222" distance of L1.end L5.end
  measures "d223" distance of L6.end L7.end
  measures "d224" distance of L6.start L8.end
  measures "d225" diameter of A3
  measures "d226" diameter of A4
  measures "d227" diameter of A5
  measures "d228" diameter of A6
extrude "Extrude60" cut sketch "Sketch25" against normal blind 36 contours L6 L7 A5 | L6 L7 A5 | L6 L8 A6 | L6 L8 A6 bodies 5
sketch "Sketch26" plane through (0, 57, 0) normal (0, -1, 0) x (1, 0, 0)
  circle A0 centre (-173.5, -7) radius 2
  circle A1 centre (-147, -7) radius 2
  circle A2 centre (-160.25, 4) radius 4.2
  circle A3 centre (-177.5, 4) radius 4.2
  circle A4 centre (-143, 4) radius 4.2
  line L0 (-137, 10) -> (-183.5, 10)
  line L1 (-183.5, 10) -> (-183.5, -12)
  line L2 (-183.5, -12) -> (-137, -12)
  line L3 (-137, -12) -> (-137, 10)
  line L4 (-137, -12) -> (-183.5, -12)
  line L5 (-183.5, -12) -> (-183.5, -2)
  line L6 (-183.5, -2) -> (-137, -2)
  line L7 (-137, -2) -> (-137, -12)
  dimension "d231" = 10
  constraint horizontal L4
  constraint vertical L5
  constraint horizontal L6
  constraint vertical L7
  constraint coincident L2.end L3.start
  measures "d231" distance of L2.end L6.end
extrude "Extrude61" add sketch "Sketch26" along normal blind 2 contours L1 L2 L3 L4 L5 L6 L7 bodies 5
sketch "Sketch27" plane through (0, 30, 0) normal (0, 1, 0) x (-1, 0, 0)
  circle A0 centre (173.5, -7) radius 2
  circle A1 centre (147, -7) radius 2
  circle A2 centre (160.25, 4) radius 4.2
  circle A3 centre (177.5, 4) radius 4.2
  circle A4 centre (143, 4) radius 4.2
  line L0 (183.5, 10) -> (137, 10)
  line L1 (137, 10) -> (137, -12)
  line L2 (137, -12) -> (183.5, -12)
  line L3 (183.5, -12) -> (183.5, 10)
  line L4 (137, -12) -> (183.5, -12)
  line L5 (183.5, -12) -> (183.5, -2)
  line L6 (183.5, -2) -> (137, -2)
  line L7 (137, -2) -> (137, -12)
  point P0 (183.5, -2)
  constraint horizontal L4
  constraint vertical L5
  constraint horizontal L6
  constraint vertical L7
  constraint coincident P0 L5.end
  constraint coincident L1.end L2.start
extrude "Extrude62" add sketch "Sketch27" along normal blind 2 contours L1 L2 L3 L4 L5 L6 L7 bodies 5
extrude "Extrude63" cut 1 faces at (-168, 57, -12) along direction (0, 0, 1) blind 10 on bodies 5 bodies 5
extrude "Extrude64" cut 2 faces at (-152.5, 30.6667, -12) (-152.5, 29.3333, -12) along direction (0, 0, 1) blind 10 on bodies 5 bodies 5
sketch "Sketch28" plane through (0, 58, 0) normal (0, 1, 0) x (-1, 0, 0)
  line L0 (137, -2) -> (183.5, -2)
  line L1 (183.5, -2) -> (183.5, 13)
  line L2 (183.5, 13) -> (137, 13)
  line L3 (137, 13) -> (137, -2)
  circle A0 centre (160.25, 4) radius 4.2
  circle A1 centre (177.5, 4) radius 4.2
  circle A2 centre (143, 4) radius 4.2
  circle A3 centre (177.5, 4) radius 4.15
  circle A4 centre (160.25, 4) radius 4.15
  circle A5 centre (143, 4) radius 4.15
  dimension "d242" = 8.3
  dimension "d243" = 8.3
  dimension "d244" = 8.3
  constraint concentric A1 A3
  constraint concentric A0 A4
  constraint concentric A2 A5
  measures "d242" diameter of A3
  measures "d243" diameter of A4
  measures "d244" diameter of A5
extrude "Extrude66" add sketch "Sketch28" against normal blind 29 contours A0 | A1 | A2 bodies 5
extrude "Extrude65" add 1 faces at (-160.3546, 57, 9.3961) along direction (0, -1, 0) blind 27 on bodies 5 bodies 5
sketch "Sketch29" plane through (0, 58, 0) normal (0, 1, 0) x (-1, 0, 0)
  circle A0 centre (177.5, 4) radius 4.15
  circle A1 centre (160.25, 4) radius 4.15
  circle A2 centre (143, 4) radius 4.15
  line L0 (137, -2) -> (183.5, -2)
  line L1 (183.5, -2) -> (183.5, 13)
  line L2 (183.5, 13) -> (137, 13)
  line L3 (137, 13) -> (137, -2)
  line L4 (183.5, -2) -> (137, -2)
  line L5 (137, -2) -> (137, 4)
  line L6 (137, 4) -> (183.5, 4)
  line L7 (183.5, 4) -> (183.5, -2)
  constraint horizontal L4
  constraint vertical L5
  constraint horizontal L6
  constraint vertical L7
  constraint coincident L3 L5.end
  constraint coincident L0.end L1.start
extrude "Extrude67" cut sketch "Sketch29" against normal blind 29 contours A0 A1 A2 L0 L1 L3 L4 L5 L6 L7 | A0 L6 | A1 L6 | A2 L6 picked at (176.2382, 3.1936) picked at (161.4203, 1.5698) picked at (144.1703, 1.5698) bodies 5
extrude "Extrude68" add sketch "Sketch29" against normal blind 29 separate body contours A0 A1 A2 L0 L1 L3 L4 L5 L6 L7 makes body 8
move_body "Move1" bodies 8 to x (1, 0, 0) y (0, 1, 0) z (0, 0, 1) at (0, 0, -5)
sketch "Sketch30" plane through (0, 58, 0) normal (0, 1, 0) x (-1, 0, 0)
  line L0 (181.65, 4) -> (183.5, 4)
  line L1 (183.5, 4) -> (183.5, 13)
  line L2 (183.5, 13) -> (137, 13)
  line L3 (137, 13) -> (137, 4)
  line L4 (137, 4) -> (138.85, 4)
  arc A0 (147.15, 4) -> (138.85, 4) centre (143, 4) ccw
  line L5 (147.15, 4) -> (156.1, 4)
  arc A1 (164.4, 4) -> (156.1, 4) centre (160.25, 4) ccw
  line L6 (164.4, 4) -> (173.35, 4)
  arc A2 (181.65, 4) -> (173.35, 4) centre (177.5, 4) ccw
  line L7 (169, 4) -> (169, 7)
  line L8 (169, 7) -> (174.35, 7)
  line L9 (174.35, 7) -> (174.35, 10.3)
  line L10 (174.35, 10.3) -> (169, 10.3)
  line L11 (169, 10.3) -> (169, 7)
  line L12 (169, 7) -> (163.65, 7)
  line L13 (163.65, 7) -> (163.65, 10.3)
  line L14 (163.65, 10.3) -> (169, 10.3)
  line L15 (169, 10.3) -> (169, 7)
  dimension "d251" = 3
  dimension "d252" = 3.3
  dimension "d253" = 5.35
  constraint vertical L7
  constraint horizontal L8
  constraint vertical L9
  constraint horizontal L10
  constraint vertical L11
  constraint horizontal L12
  constraint vertical L13
  constraint horizontal L14
  constraint vertical L15
  measures "d251" distance of L7.start L7.end
  measures "d252" distance of L7.end L10.end
  measures "d253" distance of L7.end L8.end
extrude "Extrude69" cut sketch "Sketch30" against normal blind 10 contours L8 L9 L10 L11 L15 | L11 L12 L13 L14 L15 bodies 5